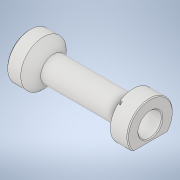
# Autodesk Inventor part: bobina_v2
Saved by Autodesk Inventor 2020 (Build 240168000, 168)
## iProperties
Part Number: bobina_v2
Material: PC/ABS-Kunststoff
Document SubType Name: Modeling
Designer: rYan
Mass: 0.662831 g
Surface Area: 50.1167 cm^2
Volume: 1.85525 cm^3
Density: 0.357273 g/cm^3
Appearance: Glatt - weiß
Author: rYan
Autodesk Inventor part; units mm, degrees
ref_plane "YZ Plane" through (0, 0, 0) normal (1, 0, 0) x (0, 1, 0)
sketch "Skizze1" plane through (0, 0, 0) normal (0, 0, 1) x (1, 0, 0)
  line L0 (-27, 0) -> (27, 0)
  line L1 (27.9, 5.4) -> (27.9, 10.5)
  line L2 (27.9, 10.5) -> (19.9, 10.5)
  line L3 (19.9, 10.5) -> (19.9, 5.9)
  line L4 (19.9, 5.9) -> (-16.9, 5.9)
  line L5 (-16.9, 5.9) -> (-21.5, 10.5)
  line L6 (-21.5, 10.5) -> (-27.9, 10.5)
  line L7 (-27.9, 10.5) -> (-27.9, 5.4)
  line L8 (0, 12.6) -> (0, -2.1) projected
  line L9 (-27.9, 5.4) -> (27.9, 5.4)
  point P0 (0, 0)
  point P1 (0, 0)
  dimension "d6" = 10.8
  dimension "d8" = 21
  dimension "d28" = 0.5
  dimension "d33" = 55.8
  dimension "d34" = 8
  dimension "d35" = 45
  dimension "d36" = 36.8
  constraints: 18 end point, 4 perpendicular, 2 point on line, 1 coincident, 1 horizontal, 1 midpoint, 2 other
  measures "d6" diameter of L9 L0
  measures "d8" diameter of L2 L0
  measures "d28" distance between parallel lines of L9 L4
  measures "d33" distance between parallel lines of L1 L7
  measures "d34" distance of L1.end L2.end
  measures "d35" angle of L5 L4
  measures "d36" distance from line of L3 L4.end
revolve "Umdrehung1" add sketch "Skizze1" angle 360 about axis through (-27, 0, 0) along (1, 0, 0)
chamfer "Fase1" distance 0.4 angle 45 4 edges at (-27.9, -5.4, 0) (27.9, -5.4, 0) (-27.9, -10.5, 0) (27.9, -10.5, 0)
ref_plane "Arbeitsebene1" through (1.5, 5.9, 0) normal (0, 1, 0) x (-1, 0, 0)
ref_plane "Arbeitsebene2" through (1.5, 6, 0) normal (0, 1, 0) x (-1, 0, 0)
sketch "Skizze2" plane through (1.5, 6, 0) normal (0, 1, 0) x (-1, 0, 0)
  line L0 (23, 10.5) -> (23, -10.5) projected
  line L1 (23, 0) -> (24, 0)
  line L2 (24, 0) -> (24, 10.5)
  line L3 (24, 10.5) -> (23, 10.5)
  line L4 (23, 10.5) -> (23, 0)
  point P0 (1.5, 0)
  point P1 (28, 10.5)
  point P2 (28, -10.5)
  dimension "d12" = 1
  constraints: 8 end point, 2 parallel, 1 horizontal, 1 midpoint, 1 perpendicular
  measures "d12" distance of L0.start L2.end
extrude "Extrusion1" [suppressed]
mirror "Spiegeln2" [suppressed]
fillet "Rundung1" [suppressed]
ref_plane "Arbeitsebene3" through (0, 0, -8.6) normal (0, 0, 1) x (1, 0, 0)
sketch "Skizze3" plane through (0, 0, -8.6) normal (0, 0, 1) x (1, 0, 0)
  line L0 (19.9, -10.5) -> (19.9, 10.5) projected
  line L1 (27.5, -10.5) -> (27.5, 10.5) projected
  line L2 (-27.5, 10.5) -> (-27.5, -10.5) projected
  line L3 (-27.9, 5.8) -> (-27.9, -5.8) projected
  line L4 (-27.9, -10.1) -> (-27.9, 10.1) projected
  line L5 (27.9, 10.1) -> (27.9, -10.1) projected
  line L6 (20.9, 10.5) -> (27.9, 10.5)
  line L7 (27.9, 10.5) -> (27.9, -10.5)
  line L8 (27.9, -10.5) -> (20.9, -10.5)
  line L9 (20.9, -10.5) -> (20.9, 10.5)
  line L10 (-27.9, 10.5) -> (-24.9, 10.5)
  line L11 (-24.9, 10.5) -> (-24.9, -10.5)
  line L12 (-24.9, -10.5) -> (-27.9, -10.5)
  line L13 (-27.9, -10.5) -> (-27.9, 10.5)
  point P0 (-25.9, -10.5)
  point P1 (-25.9, 10.5)
  dimension "d23" = 7
  dimension "d24" = 3
  constraints: 16 end point, 6 point on line, 4 parallel, 2 horizontal, 2 perpendicular
  measures "d23" distance of L7.end L8.end
  measures "d24" distance of L11.end L12.end
extrude "Extrusion2" cut sketch "Skizze3" along normal blind 2.1 and the other way blind 2.1
chamfer "Fase3" [suppressed]
chamfer "Fase4" distance 3.99 angle 45 1 edges at (20.9, 0, -6.5)
sketch "Skizze4" plane through (0, 0, 0) normal (0, 0, 1) x (1, 0, 0)
  line L0 (-21.5, 10.5) -> (-16.9, 5.9) projected
  line L1 (-27.5, 10.5) -> (-21.5, 10.5) projected
  line L2 (-24.5, 10.5) -> (-19.9, 5.9)
  line L3 (-19.9, 5.9) -> (-16.9, 5.9)
  line L4 (-33, 0) -> (5.5, 0) projected
  point P0 (0, 0)
  dimension "d37" = 3
  constraints: 4 end point, 1 horizontal, 1 midpoint, 1 parallel
  measures "d37" distance of L2.end L0.end
revolve "Umdrehung2" [suppressed]
pattern_circular "Runde Anordnung1" [suppressed]
sketch "Skizze5" plane through (19.9, 0, 0) normal (-1, 0, 0) x (0, 0, 1)
  arc A0 (-6.5, -8.2462) -> (-6.5, 8.2462) centre (0, 0) ccw projected
  line L0 (8.6856, -5.9) -> (0, -5.9)
  line L1 (0, -5.9) -> (0, -6.9)
  line L2 (0, -6.9) -> (8.6856, -6.9)
  line L3 (8.6856, -6.9) -> (8.6856, -5.9)
  circle A1 centre (0, 0) radius 5.9 projected
  point P0 (0, 0)
  point P1 (-8.6, 6.0241)
  point P2 (-8.6, -6.0241)
  dimension "d42" = 1
  constraints: 8 end point, 2 parallel, 1 horizontal, 1 perpendicular, 1 point on circle, 1 point on line, 1 tangent
  measures "d42" distance of L2.end L0.start
extrude "Extrusion3" cut sketch "Skizze5" against normal blind 1 contours L2 L1 L0 A0 | A0 L3 L2
fillet "Rundung2" radius 2 2 edges at (19.9, -6.4, 0) (20.9, -6.4, 0)
sketch "Skizze7" plane through (0, 0, 0) normal (1, 0, 0) x (0, 1, 0)
  line L0 (-11.2, 0) -> (11.2, 0) projected
  line L1 (0, 11.2) -> (0, -11.2) projected
  point P0 (0, 0)
  point P1 (-8, 0)
  point P2 (8, 0)
  dimension "d46" = 8
  constraints: 2 point on line, 1 symmetric about line
  measures "d46" distance from line of L1 point (-8, 0)
hole "Bohrung1" [suppressed]
